Autodesk Fusion 360 part; units mm, degrees
(part 2 of 3)
sketch "Sketch17" plane through (0, 0, 0) normal (0, 0, -1) x (-1, 0, 0)
  line L0 (-9.2, 0) -> (-9.2, 7.7)
  line L1 (-9.2, 7.7) -> (-13.4, 7.7)
  line L2 (-13.4, 7.7) -> (-13.4, 11.7)
  line L3 (-13.4, 11.7) -> (-21.95, 11.7)
  line L4 (-21.95, 11.7) -> (-21.95, 22.7)
  line L5 (-21.95, 22.7) -> (-13.4, 22.7)
  line L6 (-13.4, 22.7) -> (-13.4, 26.7)
  line L7 (-13.4, 26.7) -> (-9.2, 26.7)
  line L8 (-9.2, 26.7) -> (-9.2, 34.0142)
  arc A0 (-9.2, 36.3358) -> (-9.2, 34.0142) centre (-8.25, 35.175) ccw
  line L9 (-9.2, 36.3358) -> (-9.2, 43.65)
  line L10 (-9.2, 43.65) -> (-13.4, 43.65)
  line L11 (-13.4, 43.65) -> (-13.4, 47.65)
  line L12 (-13.4, 47.65) -> (-30.5, 47.65)
  line L13 (-30.5, 47.65) -> (-30.5, 34.2)
  line L14 (-30.5, 34.2) -> (-61.05, 34.2)
  line L15 (-61.05, 34.2) -> (-61.05, 32.85)
  line L16 (-61.05, 32.85) -> (-40.3, 32.85)
  line L17 (-40.3, 32.85) -> (-40.3, 1.8)
  line L18 (-40.3, 1.8) -> (-97.3, 1.8)
  line L19 (-97.3, 1.8) -> (-97.3, 8.3)
  line L20 (-97.3, 8.3) -> (-99.3, 8.3)
  line L21 (-99.3, 8.3) -> (-99.3, 1.6)
  line L22 (-99.3, 1.6) -> (-109.65, 1.6)
  line L23 (-109.65, 1.6) -> (-109.65, 34.9)
  line L24 (-109.65, 34.9) -> (-111.4, 34.9)
  line L25 (-111.4, 34.9) -> (-111.4, 0)
  line L26 (-111.4, 0) -> (-9.2, 0)
  circle A1 centre (-22.85, 35.175) radius 1.1
  line L27 (-45.8, 8.3) -> (-45.8, 26.1)
  line L28 (-45.8, 26.1) -> (-30.8, 26.1)
  line L29 (-30.8, 26.1) -> (-30.8, 8.3)
  line L30 (-30.8, 8.3) -> (-45.8, 8.3)
  line L31 (-45.8, 8.3) -> (-45.8, 26.1)
  line L32 (0, 0) -> (0, 71.5)
  line L33 (-21.95, 22.7) -> (-30.8, 22.7)
  line L34 (-21.95, 11.7) -> (-30.8, 11.7)
  line L35 (-23.45, 22.7) -> (-23.45, 11.7)
  line L36 (-29.3, 22.7) -> (-29.3, 11.7)
  line L37 (-30.8, 22.7) -> (-30.8, 11.7)
  circle A2 centre (-22.85, 35.175) radius 3.2
  line L38 (-29.3, 22.7) -> (-29.3, 46.05)
  line L39 (-29.3, 46.05) -> (-15, 46.05)
  line L40 (-15, 46.05) -> (-15, 42.05)
  line L41 (-15, 42.05) -> (-6.75, 42.05)
  line L42 (-6.75, 42.05) -> (-6.75, 46.05)
  line L43 (-6.75, 46.05) -> (-1.95, 46.05)
  line L44 (-1.95, 46.05) -> (-1.95, 23.9)
  line L45 (-1.95, 23.9) -> (-6.75, 23.9)
  line L46 (-6.75, 23.9) -> (-6.75, 27.9)
  line L47 (-6.75, 27.9) -> (-15, 27.9)
  line L48 (-15, 27.9) -> (-15, 23.9)
  line L49 (-15, 23.9) -> (-29.3, 23.9)
  line L50 (-1.95, 58.65) -> (-1.95, 47.65)
  line L51 (-23.2, 38.3558) -> (-22.5, 38.3558)
  line L52 (-22.5, 38.3558) -> (-22.5, 46.05)
  line L53 (-22.5, 46.05) -> (-23.2, 46.05)
  line L54 (-23.2, 46.05) -> (-23.2, 38.3558)
  line L55 (-23.2, 31.9942) -> (-22.5, 31.9942)
  line L56 (-22.5, 31.9942) -> (-22.5, 23.9)
  line L57 (-22.5, 23.9) -> (-23.2, 23.9)
  line L58 (-23.2, 23.9) -> (-23.2, 31.9942)
  circle A3 centre (-8.2846, 35.2649) radius 5.75
  line L59 (-6.1095, 29.9421) -> (-6.75, 27.9)
  line L60 (-10.3878, 29.9134) -> (-11.0193, 27.9)
  line L61 (-6.2019, 40.6244) -> (-6.75, 42.05)
  line L62 (-10.4655, 40.5852) -> (-11.0287, 42.05)
  circle A4 centre (-68.565, 29.235) radius 1.2
  circle A5 centre (-57.165, 29.235) radius 1.2
  circle A6 centre (-68.565, 29.235) radius 3.25
  circle A7 centre (-57.165, 29.235) radius 3.25
  line L63 (-92.05, 32.85) -> (-65.05, 32.85)
  line L64 (-61.05, 32.85) -> (-40.3, 32.85)
  line L65 (-90.75, 27.4) -> (-79.3, 27.4)
  line L66 (-79.3, 27.4) -> (-79.3, 32.85)
  line L67 (-79.3, 32.85) -> (-90.75, 32.85)
  line L68 (-90.75, 32.85) -> (-90.75, 27.4)
  line L69 (-78, 32.85) -> (-67.25, 32.85)
  line L70 (-67.25, 32.85) -> (-67.25, 27.4)
  line L71 (-67.25, 27.4) -> (-78, 27.4)
  line L72 (-78, 27.4) -> (-78, 32.85)
  line L73 (-92.05, 32.85) -> (-92.05, 26.1)
  line L74 (-92.05, 26.1) -> (-65.05, 26.1)
  line L75 (-65.05, 26.1) -> (-65.05, 32.85)
  line L76 (-40.3, 32.85) -> (-45.225, 32.85)
  line L77 (-45.225, 32.85) -> (-45.225, 27.4)
  line L78 (-45.225, 27.4) -> (-40.3, 27.4)
  line L79 (-40.3, 27.4) -> (-40.3, 32.85)
  line L80 (-46.325, 32.85) -> (-58.85, 32.85)
  line L81 (-58.85, 32.85) -> (-58.85, 27.4)
  line L82 (-58.85, 27.4) -> (-46.325, 27.4)
  line L83 (-46.325, 27.4) -> (-46.325, 32.85)
  line L84 (-65.05, 34.2) -> (-92.05, 34.2)
  line L85 (-30.5, 34.2) -> (-61.05, 34.2)
  line L86 (-61.05, 93.5) -> (-61.05, 34.2)
  line L87 (-65.05, 34.2) -> (-65.05, 93.5)
  line L88 (-92.05, 93.5) -> (-92.05, 34.2)
  line L89 (-61.05, 93.5) -> (-61.05, 34.2)
  line L90 (-61.05, 34.2) -> (-30.5, 34.2)
  line L91 (-30.5, 34.2) -> (-30.5, 47.65)
  line L92 (-30.5, 47.65) -> (-21.95, 47.65)
  line L93 (-21.95, 47.65) -> (-21.95, 58.65)
  line L94 (-21.95, 58.65) -> (-30.5, 58.65)
  line L95 (-30.5, 58.65) -> (-30.5, 93.5)
  line L96 (-30.5, 93.5) -> (-61.05, 93.5)
  line L97 (-65.05, 34.2) -> (-65.05, 93.5)
  line L98 (-65.05, 93.5) -> (-92.05, 93.5)
  line L99 (-92.05, 93.5) -> (-92.05, 34.2)
  line L100 (-92.05, 34.2) -> (-65.05, 34.2)
  line L101 (-90.95, 81.5) -> (-79.1, 81.5)
  line L102 (-79.1, 81.5) -> (-79.1, 58.4)
  line L103 (-79.1, 58.4) -> (-90.95, 58.4)
  line L104 (-90.95, 58.4) -> (-90.95, 81.5)
  line L105 (-78, 81.5) -> (-66.15, 81.5)
  line L106 (-66.15, 81.5) -> (-66.15, 58.4)
  line L107 (-66.15, 58.4) -> (-78, 58.4)
  line L108 (-78, 58.4) -> (-78, 81.5)
  line L109 (-90.95, 57.3) -> (-79.1, 57.3)
  line L110 (-79.1, 57.3) -> (-79.1, 34.2)
  line L111 (-79.1, 34.2) -> (-90.95, 34.2)
  line L112 (-90.95, 34.2) -> (-90.95, 57.3)
  line L113 (-78, 57.3) -> (-66.15, 57.3)
  line L114 (-66.15, 57.3) -> (-66.15, 34.2)
  line L115 (-66.15, 34.2) -> (-78, 34.2)
  line L116 (-78, 34.2) -> (-78, 57.3)
  line L117 (-59.95, 81.5) -> (-46.325, 81.5)
  line L118 (-46.325, 81.5) -> (-46.325, 58.4)
  line L119 (-46.325, 58.4) -> (-59.95, 58.4)
  line L120 (-59.95, 58.4) -> (-59.95, 81.5)
  line L121 (-45.225, 81.5) -> (-30.5, 81.5)
  line L122 (-30.5, 81.5) -> (-30.5, 58.4)
  line L123 (-30.5, 58.4) -> (-45.225, 58.4)
  line L124 (-45.225, 58.4) -> (-45.225, 81.5)
  line L125 (-59.95, 57.3) -> (-46.325, 57.3)
  line L126 (-46.325, 57.3) -> (-46.325, 34.2)
  line L127 (-46.325, 34.2) -> (-59.95, 34.2)
  line L128 (-59.95, 34.2) -> (-59.95, 57.3)
  line L129 (-45.225, 34.2) -> (-45.225, 57.3)
  line L130 (-45.225, 57.3) -> (-30.5, 57.3)
  line L131 (-30.5, 57.3) -> (-30.5, 47.65)
  line L132 (-30.5, 34.2) -> (-30.5, 27.2)
  line L133 (-30.5, 27.2) -> (-39.2, 27.2)
  line L134 (-39.2, 27.2) -> (-39.2, 34.2)
  line L135 (-45.225, 57.3) -> (-46.325, 57.3) construction
  line L136 (-29.3, 58.65) -> (-29.3, 47.65)
  line L137 (-22.85, 58.65) -> (-22.85, 47.65)
  line L138 (-45.7978, 81.5) -> (-45.775, 34.2) construction
  line L139 (-59.95, 57.3) -> (-59.95, 58.4) construction
  line L140 (-29.4, 60.45) -> (-29.4, 70)
  line L141 (-29.4, 70) -> (-15.05, 70)
  line L142 (-15.05, 70) -> (-15.05, 60.45)
  line L143 (-15.05, 60.45) -> (-29.4, 60.45)
  line L144 (-14.05, 70) -> (-1.7, 70)
  line L145 (-6.7, 64.45) -> (-14.05, 64.45)
  line L146 (-14.05, 64.45) -> (-14.05, 70)
  line L147 (-8.35, 62.65) -> (-8.35, 58.65)
  line L148 (-9.2, 62.65) -> (-9.2, 93.5)
  line L149 (-9.2, 93.5) -> (-30.5, 93.5)
  line L150 (-30.5, 93.5) -> (-30.5, 58.65)
  line L151 (-30.5, 58.65) -> (-13.4, 58.65)
  line L152 (-13.4, 58.65) -> (-13.4, 62.65)
  line L153 (-13.4, 62.65) -> (-9.2, 62.65)
  line L154 (-9.2, 62.65) -> (-8.35, 62.65)
  line L155 (-13.4, 58.65) -> (-13.4, 62.65)
  line L156 (-1.7, 70) -> (-1.7, 60.45)
  line L157 (-1.7, 60.45) -> (-6.7, 60.45)
  line L158 (-6, 71.5) -> (-6, 93.5)
  line L159 (0, 71.5) -> (-6, 71.5)
  line L160 (-29.4, 71.5) -> (-29.4, 81.5)
  line L161 (-29.4, 81.5) -> (-19.05, 81.5)
  line L162 (-19.05, 81.5) -> (-19.05, 71.5)
  line L163 (-19.05, 71.5) -> (-29.4, 71.5)
  line L164 (-18.05, 81.5) -> (-18.05, 71.5)
  line L165 (-18.05, 71.5) -> (-7.7, 71.5)
  line L166 (-7.7, 71.5) -> (-7.7, 81.5)
  line L167 (-7.7, 81.5) -> (-18.05, 81.5)
  line L168 (-6.7, 64.45) -> (-6.7, 60.45)
  line L169 (-98.4, 26.1) -> (-98.4, 93.5)
  line L170 (-92.05, 81.5) -> (-96.9, 81.5)
  line L171 (-96.9, 81.5) -> (-96.9, 58.4)
  line L172 (-96.9, 58.4) -> (-92.05, 58.4)
  line L173 (-92.05, 58.4) -> (-92.05, 81.5)
  line L174 (-92.05, 57.3) -> (-96.9, 57.3)
  line L175 (-96.9, 57.3) -> (-96.9, 40.9)
  line L176 (-96.9, 40.9) -> (-92.05, 40.9)
  line L177 (-92.05, 40.9) -> (-92.05, 57.3)
  line L178 (-92.05, 39.8) -> (-96.9, 39.8)
  line L179 (-96.9, 39.8) -> (-96.9, 27.4)
  line L180 (-96.9, 27.4) -> (-92.05, 27.4)
  line L181 (-92.05, 27.4) -> (-92.05, 39.8)
  line L182 (-109.65, 69.75) -> (-98.4, 69.75)
  line L183 (-98.4, 69.75) -> (-98.4, 59.45)
  line L184 (-98.4, 59.45) -> (-109.65, 59.45)
  line L185 (-109.65, 59.45) -> (-109.65, 69.75)
  line L186 (-109.65, 58.25) -> (-98.4, 58.25)
  line L187 (-98.4, 58.25) -> (-98.4, 47.95)
  line L188 (-98.4, 47.95) -> (-109.65, 47.95)
  line L189 (-109.65, 47.95) -> (-109.65, 58.25)
  circle A8 centre (-104.15, 26.7) radius 1.2
  circle A9 centre (-104.15, 26.7) radius 3.25
  circle A10 centre (-104.15, 7.7) radius 1.2
  circle A11 centre (-104.15, 7.7) radius 3.25
  line L190 (-111.4, 71.5) -> (-98.4, 71.5)
  line L191 (-109.65, 34.9) -> (-109.65, 47.95)
  line L192 (-104.5, 29.9311) -> (-103.8, 29.9311)
  line L193 (-103.8, 29.9311) -> (-103.8, 46.45)
  line L194 (-103.8, 46.45) -> (-104.5, 46.45)
  line L195 (-104.5, 46.45) -> (-104.5, 29.9311)
  line L196 (-104.5, 23.4689) -> (-103.8, 23.4689)
  line L197 (-103.8, 23.4689) -> (-103.8, 10.9311)
  line L198 (-103.8, 10.9311) -> (-104.5, 10.9311)
  line L199 (-104.5, 10.9311) -> (-104.5, 23.4689)
  line L200 (-104.5, 4.4689) -> (-103.8, 4.4689)
  line L201 (-103.8, 4.4689) -> (-103.8, 1.6)
  line L202 (-103.8, 1.6) -> (-104.5, 1.6)
  line L203 (-104.5, 1.6) -> (-104.5, 4.4689)
  line L204 (-93.55, 26.1) -> (-98.4, 26.1)
  line L205 (-97.3, 8.3) -> (-90.8, 8.3)
  line L206 (-97.3, 8.3) -> (-99.3, 8.3)
  line L207 (-93.7, 26.1) -> (-93.7, 8.3)
  line L208 (-95.5, 26.1) -> (-95.5, 17.55)
  line L209 (-95.5, 17.55) -> (-103.8, 17.55)
  line L210 (-103.8, 16.85) -> (-95.5, 16.85)
  line L211 (-95.5, 16.85) -> (-95.5, 8.3)
  line L212 (-107.3811, 27.05) -> (-109.65, 27.05)
  line L213 (-109.65, 27.05) -> (-109.65, 26.35)
  line L214 (-109.65, 26.35) -> (-107.3811, 26.35)
  line L215 (-107.3811, 26.35) -> (-107.3811, 27.05)
  line L216 (-107.3811, 8.05) -> (-109.65, 8.05)
  line L217 (-109.65, 8.05) -> (-109.65, 7.35)
  line L218 (-109.65, 7.35) -> (-107.3811, 7.35)
  line L219 (-107.3811, 7.35) -> (-107.3811, 8.05)
  line L220 (-109.65, 46.45) -> (-98.4, 46.45)
  line L221 (-59.8, 8.3) -> (-45.8, 8.3)
  line L222 (-79.1, 81.5) -> (-78, 81.5) construction
  line L223 (-30.5, 93.5) -> (-6, 93.5)
  line L224 (-6, 93.5) -> (-6, 71.5)
  line L225 (-6, 71.5) -> (-30.5, 71.5)
  line L226 (-30.5, 71.5) -> (-30.5, 93.5)
  line L227 (-103.8, 16.85) -> (-109.65, 16.85)
  line L228 (-109.65, 16.85) -> (-109.65, 17.55)
  line L229 (-109.65, 17.55) -> (-103.8, 17.55)
  line L230 (-103.8, 17.55) -> (-103.8, 16.85)
  arc A12 (-9.2, 34.0142) -> (-9.2, 36.3358) centre (-8.25, 35.175) ccw
  arc A13 (-9.2, 36.3358) -> (-9.2, 34.0142) centre (-8.25, 35.175) ccw
  circle A14 centre (-22.85, 35.175) radius 1.1
  point P0 (-45.8, 26.1)
  point P1 (-45.8, 8.3)
  point P2 (-8.35, 47.65)
  point P3 (-61.05, 26.1)
  point P4 (-61.05, 62.1271)
  point P5 (-45.775, 57.3)
  point P6 (-45.775, 93.5)
  point P7 (-59.95, 57.85)
  point P8 (-45.7864, 57.85)
  point P9 (-78.55, 81.5)
  point P10 (-78.55, 93.5)
  dimension "d197" = 30.8
  dimension "d198" = 1.5
  dimension "d199" = 1.5
  dimension "d201" = 6.4
  dimension "d202" = 1.6
  dimension "d203" = 1.6
  dimension "d204" = 1.6
  dimension "d205" = 1.6
  dimension "d206" = 1.6
  dimension "d207" = 1.2
  dimension "d208" = 0.7
  dimension "d209" = 11.5
  dimension "d210" = 6.5
  dimension "d211" = 1.3
  dimension "d212" = 1.3
  dimension "d213" = 1.3
  dimension "d214" = 2.2
  dimension "d216" = 2.2
  dimension "d217" = 1.3
  dimension "d221" = 1.1
  dimension "d222" = 1.1
  dimension "d223" = 1.1
  dimension "d224" = 1.1
  dimension "d226" = 1.1
  dimension "d227" = 1.1
  dimension "d228" = 1.1
  dimension "d229" = 1.1
  dimension "d230" = 1.1
  dimension "d231" = 1.1
  dimension "d233" = 1.1
  dimension "d234" = 0.9
  dimension "d235" = 1.2
  dimension "d236" = 1.1
  dimension "d237" = 1.7
  dimension "d238" = 1
  dimension "d239" = 1.5
  dimension "d240" = 1.8
  dimension "d242" = 1
  dimension "d243" = 1.8
  dimension "d244" = 1.65
  dimension "d245" = 1.65
  dimension "d246" = 1.7
  dimension "d247" = 1.5
  dimension "d248" = 16.4
  dimension "d249" = 1.1
  dimension "d250" = 6.5
  dimension "d251" = 6.5
  dimension "d252" = 1.2
  dimension "d253" = 10.3
  dimension "d254" = 1.75
  dimension "d255" = 0.7
  dimension "d256" = 0.7
  dimension "d257" = 0.7
  dimension "d258" = 0.7
  dimension "d259" = 1.8
  dimension "d260" = 0.7
  dimension "d261" = 1.5
  dimension "d274" = 12
  constraint horizontal L28
  constraint vertical L29
  constraint horizontal L30
  constraint vertical L31
  constraint coincident P0 L27.end
  constraint coincident L29 L33.end
  constraint perpendicular L29 L33
  constraint coincident L29 L34.end
  constraint perpendicular L29 L34
  constraint coincident L33 L35.start
  constraint coincident L34 L35.end
  constraint perpendicular L34 L35
  constraint coincident L33 L36.start
  constraint coincident L34 L36.end
  constraint perpendicular L34 L36
  constraint coincident L33 L37.start
  constraint coincident L34 L37.end
  constraint perpendicular L34 L37
  constraint collinear L29 L37
  constraint perpendicular L33 L38
  constraint perpendicular L38 L39
  constraint perpendicular L39 L40
  constraint perpendicular L9 L41
  constraint perpendicular L41 L42
  constraint perpendicular L42 L43
  constraint perpendicular L43 L44
  constraint perpendicular L44 L45
  constraint perpendicular L45 L46
  constraint perpendicular L46 L47
  constraint perpendicular L47 L48
  constraint coincident L38 L49.end
  constraint perpendicular L38 L49
  constraint vertical L43.end L50.end
  constraint equal L41 L47
  constraint equal L40 L48
  constraint equal L42 L46
  constraint vertical L40.end L47.end
  constraint horizontal L51
  constraint vertical L52
  constraint horizontal L53
  constraint vertical L54
  constraint coincident L39 L52.end
  constraint coincident A2 L51.start
  constraint coincident A2 L51.end
  constraint horizontal L55
  constraint vertical L56
  constraint horizontal L57
  constraint vertical L58
  constraint coincident L49 L56.end
  constraint coincident A2 L55.start
  constraint coincident A2 L55.end
  constraint equal L51 L55
  constraint coincident A3 L59.start
  constraint coincident A3 L60.start
  constraint coincident L47 L60.end
  constraint parallel L59 L60
  constraint coincident A3 L61.start
  constraint coincident A3 L62.start
  constraint coincident L41 L62.end
  constraint parallel L61 L62
  constraint concentric A4 A6
  constraint concentric A5 A7
  constraint equal A6 A7
  constraint horizontal L65
  constraint vertical L66
  constraint horizontal L67
  constraint vertical L68
  constraint coincident L63 L66.end
  constraint horizontal L69
  constraint vertical L70
  constraint horizontal L71
  constraint vertical L72
  constraint coincident L63 L69.start
  constraint horizontal L65.end L71.end
  constraint horizontal L76
  constraint vertical L77
  constraint horizontal L78
  constraint vertical L79
  constraint coincident L16 L17.start
  constraint horizontal L80
  constraint vertical L81
  constraint horizontal L82
  constraint vertical L83
  constraint coincident L64 L80.start
  constraint horizontal L77.end L82.end
  constraint horizontal L101
  constraint vertical L102
  constraint horizontal L103
  constraint vertical L104
  constraint horizontal L105
  constraint vertical L106
  constraint horizontal L107
  constraint vertical L108
  constraint horizontal L109
  constraint vertical L110
  constraint horizontal L111
  constraint vertical L112
  constraint horizontal L113
  constraint vertical L114
  constraint horizontal L115
  constraint vertical L116
  constraint vertical L103.end L109.start
  constraint horizontal L102.end L107.end
  constraint vertical L102.end L109.end
  constraint vertical L107.end L113.start
  constraint horizontal L117
  constraint vertical L118
  constraint horizontal L119
  constraint vertical L120
  constraint horizontal L121
  constraint vertical L122
  constraint horizontal L123
  constraint vertical L124
  constraint horizontal L125
  constraint vertical L126
  constraint horizontal L127
  constraint vertical L128
  constraint collinear L95 L122
  constraint collinear L14 L127
  constraint coincident L85 L129.start
  constraint perpendicular L125 L129
  constraint perpendicular L95 L130
  constraint coincident L12.end L13.start
  constraint perpendicular L92 L131
  constraint coincident L13.end L14.start
  constraint perpendicular L90 L132
  constraint perpendicular L132 L133
  constraint coincident L85 L134.end
  constraint perpendicular L85 L134
  constraint horizontal L117.start L121.end
  constraint horizontal L125.end L130.end
  constraint vertical L119.end L125.start
  constraint horizontal L105.end L117.start
  constraint horizontal L101.end L105.start
  constraint vertical L106.end L113.end
  constraint midpoint L135 P5
  constraint midpoint L96 P6
  constraint vertical P5 P6
  constraint horizontal L111.end L115.end
  constraint horizontal L109.start L113.end
  constraint coincident L94 L136.start
  constraint coincident L92 L136.end
  constraint perpendicular L94 L136
  constraint coincident L94 L137.start
  constraint coincident L92 L137.end
  constraint perpendicular L92 L137
  constraint midpoint L85 L138.end
  constraint midpoint L139 P7
  constraint horizontal L117.start L138.start
  constraint midpoint L138 P8
  constraint horizontal P7 P8
  constraint perpendicular L94 L140
  constraint perpendicular L136 L141
  constraint perpendicular L141 L142
  constraint perpendicular L136 L143
  constraint perpendicular L142 L144
  constraint perpendicular L142 L145
  constraint perpendicular L144 L146
  constraint perpendicular L144 L156
  constraint perpendicular L140 L161
  constraint perpendicular L160 L163
  constraint perpendicular L163 L164
  constraint perpendicular L148 L165
  constraint perpendicular L165 L166
  constraint perpendicular L164 L167
  constraint equal L161 L167
  constraint vertical L140.end L160.start
  constraint horizontal L162.end L164.end
  constraint horizontal L141.end L144.start
  constraint coincident L140.start L143.end
  constraint vertical L145.start L157.end
  constraint coincident L144.end L156.start
  constraint perpendicular L157 L168
  constraint horizontal L142.end L157.end
  constraint horizontal L170
  constraint vertical L171
  constraint horizontal L172
  constraint vertical L173
  constraint coincident L88 L170.start
  constraint horizontal L103.end L171.end
  constraint horizontal L101.start L170.start
  constraint horizontal L174
  constraint vertical L175
  constraint horizontal L176
  constraint vertical L177
  constraint coincident L88 L174.start
  constraint vertical L171.end L174.end
  constraint horizontal L178
  constraint vertical L179
  constraint horizontal L180
  constraint vertical L181
  constraint coincident L88 L178.start
  constraint horizontal L65.start L180.end
  constraint vertical L175.end L179.end
  constraint horizontal L106.end L119.end
  constraint horizontal L109.start L174.start
  constraint horizontal L182
  constraint vertical L183
  constraint horizontal L184
  constraint vertical L185
  constraint horizontal L186
  constraint vertical L187
  constraint horizontal L188
  constraint vertical L189
  constraint concentric A8 A9
  constraint concentric A10 A11
  constraint vertical L23.end L188.end
  constraint vertical L184.end L186.start
  constraint collinear L169 L183
  constraint collinear L169 L187
  constraint equal L185 L189
  constraint coincident L23.end L24.start
  constraint horizontal L192
  constraint vertical L193
  constraint horizontal L194
  constraint vertical L195
  constraint coincident A9 L192.start
  constraint coincident A9 L192.end
  constraint horizontal L196
  constraint vertical L197
  constraint horizontal L198
  constraint vertical L199
  constraint coincident A11 L197.end
  constraint coincident A9 L196.start
  constraint coincident A11 L198.end
  constraint horizontal L200
  constraint vertical L201
  constraint horizontal L202
  constraint vertical L203
  constraint coincident L22 L201.end
  constraint coincident A11 L200.start
  constraint coincident A11 L200.end
  constraint coincident L204 L208.start
  constraint perpendicular L204 L208
  constraint coincident L197 L209.end
  constraint perpendicular L197 L209
  constraint coincident L197 L210.start
  constraint perpendicular L207 L210
  constraint coincident L205 L211.end
  constraint perpendicular L205 L211
  constraint equal L208 L211
  constraint vertical L208.end L210.end
  constraint horizontal L212
  constraint vertical L213
  constraint horizontal L214
  constraint vertical L215
  constraint coincident L23 L213.end
  constraint coincident A9 L212.start
  constraint coincident A9 L214.end
  constraint horizontal L216
  constraint vertical L217
  constraint horizontal L218
  constraint vertical L219
  constraint coincident L23 L217.end
  constraint coincident A11 L216.start
  constraint coincident A11 L218.end
  constraint equal L214 L216
  constraint coincident L194.end L195.start
  constraint coincident L191 L220.start
  constraint coincident L169 L220.end
  constraint perpendicular L169 L220
  constraint collinear L194 L220
  constraint collinear L30 L221
  constraint vertical L118.end L125.end
  constraint midpoint L222 P9
  constraint midpoint L98 P10
  constraint vertical P9 P10
  constraint horizontal L223
  constraint vertical L224
  constraint horizontal L225
  constraint vertical L226
  constraint coincident L95.end L96.start
  constraint horizontal L161.end L164.start
  constraint horizontal L121.end L160.end
  constraint coincident L158.end L223.end
  constraint collinear L165 L225
  constraint collinear L17 L79
  constraint vertical L80.start L126.end
  constraint vertical L76.end L129.start
  constraint vertical L69.start L115.end
  constraint horizontal L227
  constraint vertical L228
  constraint horizontal L229
  constraint vertical L230
  constraint coincident L23 L228.end
  constraint horizontal L208.end L228.end
  constraint coincident L3.end L4.start
  constraint coincident L4.end L5.start
  constraint coincident L158.start L159.end
  constraint collinear L100 L111
  measures "d197" distance of L29 L32
  measures "d198" distance of L4 L35
  measures "d199" distance of L36 L37
  measures "d201" diameter of A2
  measures "d202" distance of L43 L50.end
  measures "d203" distance of L9.end L41
  measures "d204" horizontal distance of L42.end P2
  measures "d205" distance of L11 L40
  measures "d206" distance of L12 L39
  measures "d207" distance of L33 L49
  measures "d208" distance of L52 L54
  measures "d209" diameter of A3
  measures "d210" diameter of A6
  measures "d211" distance of L68 L73
  measures "d212" distance of L65 L74
  measures "d213" distance of L66 L72
  measures "d214" distance of L70 L75
  measures "d216" distance of L15.end L81
  measures "d217" distance of L82 P3
  measures "d221" distance of L126 L129
  measures "d222" distance of L118 L124
  measures "d223" distance of L123 L130
  measures "d224" distance of L119 L125
  measures "d226" distance of L86 L128
  measures "d227" distance of L17 L134
  measures "d228" distance of L28 L133
  measures "d229" distance of L87 L114
  measures "d230" distance of L110 L116
  measures "d231" distance of L88 L112
  measures "d233" distance of L107 L113
  measures "d234" distance of L93 L137
  measures "d235" distance of L131 L136
  measures "d236" distance of L122 L160
  measures "d237" distance of L158 L166
  measures "d238" distance of L162 L164
  measures "d239" distance of L141 L163
  measures "d240" distance of L94 L143
  measures "d242" distance of L142 L146
  measures "d243" distance of L145 L153
  measures "d244" distance of L147 L168
  measures "d245" distance of L142 L152
  measures "d246" distance of L32 L156
  measures "d247" distance of L169 L179
  measures "d248" distance of L174 L176
  measures "d249" distance of L176 L178
  measures "d250" diameter of A9
  measures "d251" diameter of A11
  measures "d252" distance of L184 L186
  measures "d253" distance of L182 L184
  measures "d254" distance of L182 L190
  measures "d255" distance of L193 L195
  measures "d256" distance of L197 L199
  measures "d257" distance of L201 L203
  measures "d258" distance of L209 L210
  measures "d259" distance of L207 L208
  measures "d260" distance of L212 L214
  measures "d261" distance of L188 L220
  measures "d274" distance of L161 L223
extrude "Extrude36" cut sketch "Sketch17" against normal blind 26.15 contours L23 A9 L191 L195 L212 L220 | L23 A9 L199 L214 L229 | L169 L186 L187 L188 L189 | L169 A9 L193 L197 L204 L208 L209 L220 | L23 A11 L199 L216 L227 | L22 L23 A11 L203 L218 | L20 L21 L22 A11 L197 L201 L205 L206 L210 L211 | L16 L17 L64 L76 L77 L78 L79 | L16 A7 L64 L80 L81 L82 L83 | L14 L85 L90 L125 L126 L127 L128 | L13 L14 L85 L90 L91 L129 L130 L131 | L95 L121 L122 L123 L124 L150 L226 | L14 L85 L90 L132 L133 L134 | L148 L165 L166 L167 L225 | L148 L164 L165 L167 L225 | L160 L161 L162 L163 L225 | L144 L145 L148 L156 L157 L168 | L144 L145 L146 L148 | A6 L63 L69 L70 L71 L72 | L63 L65 L66 L67 L68 | L73 L88 L99 L178 L179 L180 L181 | L84 L100 L109 L110 L111 L112 | L88 L99 L174 L175 L176 L177 | L84 L100 L113 L114 L115 L116 | L88 L99 L170 L171 L172 L173 | L101 L102 L103 L104 | L105 L106 L107 L108 | L117 L118 L119 L120 | L140 L141 L142 L143 | L169 L182 L183 L184 L185
extrude "Extrude37" cut sketch "Sketch17" against normal blind 40.5 contours L33 L34 L35 L36 | A2 L38 L39 L49 L54 L58 | L42 L43 L44 L45 L46 A3 L59 L61 | A2 L39 L40 L41 L47 L48 L49 L52 L56 A3 L60 L62 | L12 L92 L94 L136 L137 L151
extrude "Extrude38" cut sketch "Sketch17" against normal blind 15.5 contours L8 L47 A3 L60 | L8 L47 A3 L59 | L8 A0 L9 A3 A13 | L8 L9 A3 A12 | A0 A12 A13 | L9 L41 A3 L62 | L9 L41 A3 L61
extrude "Extrude39" cut sketch "Sketch17" against normal blind 19 contours L17 L28 L29 L30 L37 | L17 L27 L28 L30 L31
extrude "Extrude40" cut sketch "Sketch17" against normal blind 15 contours L29 L33 L34 L36 L37
extrude "Extrude41" cut sketch "Sketch17" against normal blind 11.6 contours L4 L33 L34 L35
extrude "Extrude42" cut sketch "Sketch17" against normal up to surface (4.5 mm away) contours L95 L122 L148 L149 L150 L160 L161 L162 L164 L167 L223 L225 L226 | L148 L158 L166 L167 L223 L224 L225
sketch "Sketch18" plane through (0, 93.5, 0) normal (0, 1, 0) x (-1, 0, 0)
  circle A0 centre (-78, 12.2) radius 1.3
  circle A1 centre (-46.1, 25.7) radius 1.3
  circle A2 centre (-22.7, 25.7) radius 1.3
  line L0 (-61.05, 4.5) -> (-6, 4.5)
  line L1 (-6, 4.5) -> (-6, 42.8)
  line L2 (-6, 42.8) -> (-30.75, 42.8)
  line L3 (-30.75, 42.8) -> (-30.75, 33.3)
  line L4 (-30.75, 33.3) -> (-98.4, 33.3)
  line L5 (-98.4, 33.3) -> (-98.4, 12.55)
  line L6 (-98.4, 12.55) -> (-93.55, 12.55)
  arc A3 (-92.05, 11.05) -> (-93.55, 12.55) centre (-93.55, 11.05) ccw
  line L7 (-92.05, 11.05) -> (-92.05, 4.5)
  line L8 (-92.05, 4.5) -> (-65.05, 4.5)
  line L9 (-65.05, 4.5) -> (-65.05, 10.55)
  arc A4 (-61.05, 10.55) -> (-65.05, 10.55) centre (-63.05, 10.55) ccw
  line L10 (-61.05, 10.55) -> (-61.05, 4.5)
  circle A5 centre (-17.7, 4.5) radius 3.125
  circle A6 centre (-22.7, 25.7) radius 1.3
  circle A7 centre (-17.7, 4.5) radius 1.3
  dimension "d278" = 6.25
  dimension "d279" = 11.7
  constraint coincident L0 A5.centre
  constraint concentric A5 A7
  constraint equal A6 A7
  measures "d278" diameter of A5
  measures "d279" distance of L0.end A5.centre
extrude "Extrude43" add sketch "Sketch18" against normal up to surface (12 mm away) contours L0 A7 | L0 A5 A7 picked at (-17.4106, 3.642) picked at (-15.1998, 4.2802)
extrude "Extrude44" cut sketch "Sketch18" against normal blind 10 contours L0 A7 | L0 A7
sketch "Sketch19" plane through (1.95, 0, 0) normal (1, 0, 0) x (0, 0, -1)
  line L0 (-7.25, 23.9) -> (-7.25, 46.05)
  line L1 (-7.25, 46.05) -> (-40.5, 46.05)
  line L2 (-40.5, 46.05) -> (-40.5, 44.575)
  line L3 (-40.5, 44.575) -> (-22.4117, 44.575)
  arc A0 (-22.4117, 44.575) -> (-22.4117, 41.075) centre (-19.975, 42.825) ccw
  line L4 (-22.4117, 41.075) -> (-40.5, 41.075)
  line L5 (-40.5, 41.075) -> (-40.5, 23.9)
  line L6 (-40.5, 23.9) -> (-7.25, 23.9)
  circle A1 centre (-19.975, 42.825) radius 1.325
  line L7 (-7.25, 46.05) -> (-40.5, 46.05)
  circle A2 centre (-19.975, 42.825) radius 3.225
  line L8 (-19.975, 39.6) -> (-40.5, 39.6)
  line L9 (-40.5, 44.575) -> (-40.5, 41.075)
  line L10 (-40.5, 41.075) -> (-40.5, 23.9)
  line L11 (-40.5, 46.05) -> (-40.5, 44.575)
  constraint concentric A0 A2
  constraint tangent L1 A2
  constraint coincident A2 L8.start
  constraint coincident L5 L8.end
  constraint tangent A2 L8
  constraint perpendicular L5 L8
extrude "Extrude45" add sketch "Sketch19" along normal blind 2 contours L1 L2 L3 L7 A2 L11 | L3 A0 L4 A2 | L4 L5 A2 L8 L10 | L3 L4 A2 L9 | L3 A0 L4 A2
extrude "Extrude46" cut 1 faces at (1.95, 42.8941, 34.6559) along direction (1, 0, 0) up to surface (0.15 mm away)
fillet "Fillet2" radius 5 1 edges at (45.8, 17.2, 19)
sketch "Sketch20" plane through (0, 0, 0) normal (0, -1, 0) x (1, 0, 0)
  line L0 (0, 9.2) -> (9.2, 0)
  line L1 (111.4, 0) -> (111.4, 33.3)
  line L2 (111.4, 33.3) -> (99, 33.3)
  line L3 (99, 33.3) -> (99, 47.8)
  line L4 (99, 47.8) -> (38.2, 47.8)
  line L5 (38.2, 47.8) -> (38.2, 42.8)
  line L6 (38.2, 42.8) -> (0, 42.8)
  line L7 (0, 42.8) -> (0, 9.2)
  circle A0 centre (63.05, 41.55) radius 1.75
  circle A1 centre (78.55, 26.05) radius 12
  circle A2 centre (94.05, 41.55) radius 1.75
  line L8 (38.2, 40.8) -> (20.65, 40.8)
  line L9 (20.65, 40.8) -> (20.65, 26.8)
  line L10 (20.65, 26.8) -> (38.2, 26.8)
  line L11 (38.2, 26.8) -> (38.2, 40.8)
  line L12 (19.55, 40.8) -> (19.55, 26.8)
  line L13 (19.55, 26.8) -> (2, 26.8)
  line L14 (2, 26.8) -> (2, 40.8)
  line L15 (2, 40.8) -> (19.55, 40.8)
  line L16 (38.2, 25.7) -> (38.2, 2)
  line L17 (38.2, 2) -> (20.65, 2)
  line L18 (20.65, 2) -> (20.65, 25.7)
  line L19 (20.65, 25.7) -> (38.2, 25.7)
  line L20 (19.55, 25.7) -> (19.55, 2)
  line L21 (19.55, 2) -> (10.0284, 2)
  line L22 (10.0284, 2) -> (2, 10.0284)
  line L23 (2, 10.0284) -> (2, 25.7)
  line L24 (2, 25.7) -> (19.55, 25.7)
  circle A3 centre (78.55, 26.05) radius 13.8638
  line L25 (97.35, 45.8) -> (40.2, 45.8)
  line L26 (40.2, 45.8) -> (40.2, 4)
  line L27 (40.2, 4) -> (97.35, 4)
  line L28 (97.35, 4) -> (97.35, 45.8)
  circle A4 centre (63.05, 10.55) radius 3.25
  circle A5 centre (63.05, 41.55) radius 3.25
  circle A6 centre (94.05, 41.55) radius 3.25
  circle A7 centre (94.05, 10.55) radius 3.25
  line L29 (97.35, 25.4) -> (92.3986, 25.4)
  line L30 (92.3986, 25.4) -> (92.3986, 26.7)
  line L31 (92.3986, 26.7) -> (97.35, 26.7)
  line L32 (97.35, 26.7) -> (97.35, 25.4)
  line L33 (79.2, 12.2014) -> (77.9, 12.2014)
  line L34 (77.9, 12.2014) -> (77.9, 4)
  line L35 (77.9, 4) -> (79.2, 4)
  line L36 (79.2, 4) -> (79.2, 12.2014)
  line L37 (79.2, 39.8986) -> (77.9, 39.8986)
  line L38 (77.9, 39.8986) -> (77.9, 45.8)
  line L39 (77.9, 45.8) -> (79.2, 45.8)
  line L40 (79.2, 45.8) -> (79.2, 39.8986)
  line L41 (64.7014, 25.4) -> (40.2, 25.4)
  line L42 (40.2, 25.4) -> (40.2, 26.7)
  line L43 (40.2, 26.7) -> (64.7014, 26.7)
  line L44 (64.7014, 26.7) -> (64.7014, 25.4)
  line L45 (63.7, 44.7343) -> (62.4, 44.7343)
  line L46 (62.4, 44.7343) -> (62.4, 45.8)
  line L47 (62.4, 45.8) -> (63.7, 45.8)
  line L48 (63.7, 45.8) -> (63.7, 44.7343)
  line L49 (94.7, 44.7343) -> (93.4, 44.7343)
  line L50 (93.4, 44.7343) -> (93.4, 45.8)
  line L51 (93.4, 45.8) -> (94.7, 45.8)
  line L52 (94.7, 45.8) -> (94.7, 44.7343)
  line L53 (59.8657, 9.9) -> (40.2, 9.9)
  line L54 (40.2, 9.9) -> (40.2, 11.2)
  line L55 (40.2, 11.2) -> (59.8657, 11.2)
  line L56 (59.8657, 11.2) -> (59.8657, 9.9)
  line L57 (59.8657, 40.9) -> (40.2, 40.9)
  line L58 (40.2, 40.9) -> (40.2, 42.2)
  line L59 (40.2, 42.2) -> (59.8657, 42.2)
  line L60 (59.8657, 42.2) -> (59.8657, 40.9)
  circle A8 centre (63.05, 41.55) radius 4.7
  circle A9 centre (94.05, 41.55) radius 4.7
  circle A10 centre (94.05, 10.55) radius 4.7
  circle A11 centre (63.05, 10.55) radius 4.7
  line L61 (67.75, 41.55) -> (67.75, 45.8)
  line L62 (58.35, 41.55) -> (58.35, 45.8)
  line L63 (89.35, 41.55) -> (89.35, 45.8)
  line L64 (89.35, 10.55) -> (89.35, 4)
  line L65 (58.35, 10.55) -> (58.35, 4)
  line L66 (67.05, 8.0822) -> (67.05, 4)
  line L67 (13.55, 2) -> (13.55, 25.7) construction
  line L68 (8.2, 3.8284) -> (8.2, 25.7) construction
  line L69 (13.55, 26.8) -> (13.55, 40.8) construction
  line L70 (8.2, 26.8) -> (8.2, 40.8) construction
  line L71 (30.8, 2) -> (30.8, 25.7) construction
  line L72 (30.8, 26.8) -> (30.8, 40.8) construction
  line L73 (15.275, 2) -> (6.275, 2)
  line L74 (6.275, 2) -> (6.275, 25.7)
  line L75 (6.275, 25.7) -> (15.275, 25.7)
  line L76 (15.275, 25.7) -> (15.275, 2)
  line L77 (15.275, 26.8) -> (6.275, 26.8)
  line L78 (6.275, 26.8) -> (6.275, 40.8)
  line L79 (6.275, 40.8) -> (15.275, 40.8)
  line L80 (15.275, 40.8) -> (15.275, 26.8)
  line L81 (13.55, 33.8) -> (8.2, 33.8) construction
  line L82 (38.2, 26.8) -> (29.2, 26.8)
  line L83 (29.2, 26.8) -> (29.2, 40.8)
  line L84 (29.2, 40.8) -> (38.2, 40.8)
  line L85 (38.2, 40.8) -> (38.2, 26.8)
  line L86 (29.2, 25.7) -> (29.2, 2)
  line L87 (9.2, 0) -> (111.4, 0)
  circle A12 centre (63.05, 10.55) radius 1.75
  circle A13 centre (94.05, 10.55) radius 1.75
  point P0 (30.8, 0)
  point P1 (10.775, 26.8)
  point P2 (10.775, 40.8)
  point P3 (13.55, 12.5571)
  point P4 (8.2, 12.5571)
  dimension "d291" = 6.5
  dimension "d292" = 1.65
  dimension "d293" = 2
  dimension "d294" = 2
  dimension "d296" = 1.3
  dimension "d297" = 1.3
  dimension "d298" = 1.3
  dimension "d299" = 1.3
  dimension "d300" = 1.3
  dimension "d301" = 1.3
  dimension "d302" = 1.3
  dimension "d303" = 1.3
  dimension "d304" = 1.1
  dimension "d305" = 1.1
  dimension "d306" = 2
  dimension "d307" = 2
  dimension "d309" = 2
  dimension "d310" = 14
  dimension "d311" = 2
  dimension "d312" = 9.4
  dimension "d313" = 8.7
  dimension "d325" = 9
  constraint perpendicular L5 L8
  constraint perpendicular L8 L9
  constraint perpendicular L9 L10
  constraint perpendicular L8 L11
  constraint perpendicular L10 L12
  constraint perpendicular L9 L13
  constraint perpendicular L13 L14
  constraint perpendicular L14 L15
  constraint horizontal L8.end L12.start
  constraint perpendicular L8 L16
  constraint perpendicular L9 L17
  constraint perpendicular L10 L18
  constraint perpendicular L16 L19
  constraint perpendicular L17 L20
  constraint perpendicular L20 L21
  constraint perpendicular L21 L23
  constraint perpendicular L23 L24
  constraint vertical L13.end L23.end
  constraint vertical L12.end L20.start
  constraint horizontal L17.end L20.end
  constraint horizontal L9.end L12.end
  constraint horizontal L18.end L20.start
  constraint concentric A1 A3
  constraint horizontal L25
  constraint vertical L26
  constraint horizontal L27
  constraint vertical L28
  constraint concentric A4 A12
  constraint concentric A0 A5
  constraint concentric A2 A6
  constraint equal A4 A7
  constraint equal A6 A7
  constraint equal A5 A6
  constraint horizontal L29
  constraint vertical L30
  constraint horizontal L31
  constraint vertical L32
  constraint coincident A3 L30.end
  constraint coincident L28 L29.start
  constraint coincident A3 L29.end
  constraint horizontal L33
  constraint vertical L34
  constraint horizontal L35
  constraint vertical L36
  constraint coincident L27 L34.end
  constraint coincident A3 L33.start
  constraint horizontal L37
  constraint vertical L38
  constraint horizontal L39
  constraint vertical L40
  constraint coincident L25 L38.end
  constraint coincident A3 L37.start
  constraint coincident A3 L33.end
  constraint coincident A3 L37.end
  constraint horizontal L41
  constraint vertical L42
  constraint horizontal L43
  constraint vertical L44
  constraint coincident L26 L42.end
  constraint coincident A3 L41.start
  constraint coincident A3 L43.end
  constraint horizontal L45
  constraint vertical L46
  constraint horizontal L47
  constraint vertical L48
  constraint coincident L25 L46.end
  constraint coincident A5 L45.start
  constraint horizontal L49
  constraint vertical L50
  constraint horizontal L51
  constraint vertical L52
  constraint coincident L25 L50.end
  constraint coincident A6 L49.start
  constraint horizontal L53
  constraint vertical L54
  constraint horizontal L55
  constraint vertical L56
  constraint coincident L26 L54.end
  constraint coincident A4 L53.start
  constraint coincident A4 L55.end
  constraint coincident A5 L45.end
  constraint coincident A6 L49.end
  constraint horizontal L57
  constraint vertical L58
  constraint horizontal L59
  constraint vertical L60
  constraint coincident L26 L58.end
  constraint coincident A5 L57.start
  constraint coincident A5 L59.end
  constraint vertical L9.end L18.end
  constraint equal L19 L24
  constraint parallel L0 L22
  constraint vertical L10.end L16.start
  constraint concentric A0 A8
  constraint concentric A2 A9
  constraint concentric A7 A10
  constraint concentric A4 A11
  constraint equal A8 A11
  constraint equal A10 A11
  constraint equal A9 A10
  constraint coincident A8 L61.start
  constraint coincident L25 L61.end
  constraint tangent A8 L61
  constraint perpendicular L25 L61
  constraint coincident A8 L62.start
  constraint coincident L25 L62.end
  constraint tangent A8 L62
  constraint perpendicular L25 L62
  constraint coincident A9 L63.start
  constraint coincident L25 L63.end
  constraint tangent A9 L63
  constraint perpendicular L25 L63
  constraint coincident A10 L64.start
  constraint coincident L27 L64.end
  constraint tangent A10 L64
  constraint perpendicular L27 L64
  constraint coincident A11 L65.start
  constraint coincident L27 L65.end
  constraint tangent A11 L65
  constraint perpendicular L27 L65
  constraint coincident A11 L66.start
  constraint coincident L27 L66.end
  constraint perpendicular L27 L66
  constraint coincident L21 L67.start
  constraint coincident L24 L67.end
  constraint perpendicular L24 L67
  constraint coincident L22 L68.start
  constraint coincident L24 L68.end
  constraint perpendicular L24 L68
  constraint coincident L13 L69.start
  constraint coincident L15 L69.end
  constraint perpendicular L15 L69
  constraint coincident L13 L70.start
  constraint coincident L15 L70.end
  constraint perpendicular L15 L70
  constraint coincident L17 L71.start
  constraint coincident L19 L71.end
  constraint perpendicular L19 L71
  constraint coincident L10 L72.start
  constraint coincident L8 L72.end
  constraint perpendicular L8 L72
  constraint vertical P0 L71.start
  constraint vertical L71.end L72.start
  constraint vertical L67.end L69.start
  constraint vertical L68.end L70.start
  constraint horizontal L73
  constraint vertical L74
  constraint horizontal L75
  constraint vertical L76
  constraint coincident L24 L74.end
  constraint coincident L21 L73.start
  constraint horizontal L77
  constraint vertical L78
  constraint horizontal L79
  constraint vertical L80
  constraint coincident L15 L78.end
  constraint coincident L13 L77.start
  constraint midpoint L69 L81.start
  constraint midpoint L70 L81.end
  constraint horizontal L82
  constraint vertical L83
  constraint horizontal L84
  constraint vertical L85
  constraint coincident L8 L83.end
  constraint equal L77 L82
  constraint midpoint L77 P1
  constraint midpoint L15 P2
  constraint vertical P1 P2
  constraint vertical L75.end L77.start
  constraint vertical L74.end L77.end
  constraint coincident L19 L86.start
  constraint coincident L17 L86.end
  constraint perpendicular L17 L86
  constraint vertical L82.end L86.start
  measures "d291" diameter of A5
  measures "d292" distance of L3 L28
  measures "d293" distance of L4 L25
  measures "d294" distance of L5 L26
  measures "d296" distance of L57 L59
  measures "d297" distance of L41 L43
  measures "d298" distance of L53 L55
  measures "d299" distance of L34 L36
  measures "d300" distance of L38 L40
  measures "d301" distance of L29 L31
  measures "d302" distance of L50 L52
  measures "d303" distance of L46 L48
  measures "d304" distance of L18 L20
  measures "d305" distance of L10 L19
  measures "d306" distance of L7 L23
  measures "d307" distance of L0 L22
  measures "d309" distance of L11 L26
  measures "d310" distance of L8 L10
  measures "d311" distance of L6 L8
  measures "d312" diameter of A8
  measures "d313" distance of L65 L66
  measures "d325" distance of L78 L80
extrude "Extrude47" cut sketch "Sketch20" against normal blind 6.6 contours A3 L25 L28 L31 L40 A9 L63 | A3 L27 L28 L29 L36 A10 L64 | A3 L25 L26 L38 L43 L57 A8 L61 | A3 L26 L27 L34 L41 L55 A11 L66 | L26 L27 L53 L65 | L25 L26 L59 L62
sketch "Sketch21" plane through (0, 0, 2) normal (0, 0, -1) x (-1, 0, 0)
  line L0 (-40.3, 8.3) -> (-59.8, 8.3)
  line L1 (-59.8, 8.3) -> (-59.8, 3.4)
  line L2 (-59.8, 3.4) -> (-66.3, 3.4)
  line L3 (-66.3, 3.4) -> (-66.3, 8.3)
  line L4 (-66.3, 8.3) -> (-90.8, 8.3)
  line L5 (-90.8, 8.3) -> (-90.8, 3.4)
  line L6 (-90.8, 3.4) -> (-97.3, 3.4)
  circle A0 centre (-57.165, 5.235) radius 1.2
  circle A1 centre (-68.565, 5.235) radius 1.2
  circle A2 centre (-68.565, 5.235) radius 3.25
  circle A3 centre (-57.165, 5.235) radius 3.25
  line L7 (-97.3, 3.4) -> (-97.3, 1.8)
  line L8 (-97.3, 1.8) -> (-40.3, 1.8)
  line L9 (-40.3, 1.8) -> (-40.3, 8.3)
  dimension "d316" = 6.5
  constraint concentric A1 A2
  constraint concentric A0 A3
  constraint equal A2 A3
  measures "d316" diameter of A2
extrude "Extrude48" add sketch "Sketch21" against normal up to surface (38.9 mm away) contours L0 L1 L2 A3
extrude "Extrude49" add sketch "Sketch21" against normal blind 8 contours L2 L3 L4 A2
extrude "Extrude50" cut sketch "Sketch20" against normal blind 1.9 contours L25 L28 A6 L50 L52 A9 | L28 A10 | L25 A9 L63 | L25 L28 A9 | L27 L28 A10 L64 | L25 A8 L61 | L27 L53 A11 L65 L66 | L25 A5 L48 L57 A8 | L25 A6 L50 L51 L52 | A4 L53 L55 A11 | L25 A5 L46 L47 L48 | L25 L59 A8 L62 | L25 A5 L46 L59 A8 picked at (96.7504, 13.777) picked at (59.6818, 8.0267)
extrude "Extrude51" cut sketch "Sketch20" against normal blind 10 contours L22 L23 L24 L74 | L20 L21 L24 L76 | L8 L9 L10 L83 | L12 L13 L15 L80 | L13 L14 L15 L78 | L17 L18 L19 L86
extrude "Extrude52" cut sketch "Sketch20" against normal blind 6 contours L21 L22 L24 L73 L74 L75 L76 | L8 L10 L11 L82 L83 L84 L85 | L13 L15 L77 L78 L79 L80 | L16 L17 L19 L86